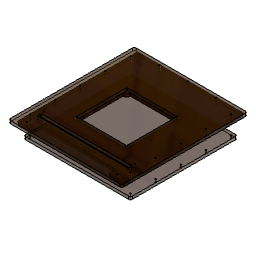
Module Plate Template (Autodesk Fusion 360 design; units mm, degrees)
Autodesk Fusion 360 part; units mm, degrees
sketch "Sketch1" plane through (0, 0, 0) normal (0, 0, 1) x (1, 0, 0)
  line L0 (-100, 0) -> (100, 0) construction
  line L1 (90, 0) -> (-90, 0)
  line L2 (-90, 0) -> (-90, 200)
  line L3 (-90, 200) -> (90, 200)
  line L4 (90, 200) -> (90, 0)
  line L5 (90, 0) -> (-90, 200) construction
  line L6 (-90, 0) -> (90, 200) construction
  line L7 (85, 0) -> (-85, 0)
  line L8 (-85, 0) -> (-85, 200)
  line L9 (-85, 200) -> (85, 200)
  line L10 (85, 200) -> (85, 0)
  line L11 (85, 0) -> (-85, 200) construction
  line L12 (-85, 0) -> (85, 200) construction
  line L13 (-60, 8) -> (-60, 21)
  line L14 (-60, 21) -> (60, 21)
  line L15 (60, 21) -> (60, 8)
  line L16 (60, 8) -> (-60, 21) construction
  line L17 (-60, 8) -> (60, 21) construction
  line L18 (-85, 8) -> (-60, 8)
  line L19 (60, 8) -> (85, 8)
  line L20 (0, 200) -> (0, 21) construction
  line L21 (40, 58) -> (-40, 58)
  line L22 (-40, 58) -> (-40, 138)
  line L23 (-40, 138) -> (40, 138)
  line L24 (40, 138) -> (40, 58)
  line L25 (40, 58) -> (-40, 138) construction
  line L26 (-40, 58) -> (40, 138) construction
  circle A0 centre (-40, 138) radius 1
  circle A1 centre (40, 138) radius 1
  circle A2 centre (-40, 58) radius 1
  circle A3 centre (40, 58) radius 1
  circle A4 centre (-40, 138) radius 6
  circle A5 centre (40, 138) radius 6
  circle A6 centre (40, 58) radius 6
  circle A7 centre (-40, 58) radius 6
  line L27 (-80, 200) -> (-80, 8) construction
  line L28 (80, 8) -> (80, 200) construction
  circle A8 centre (-80, 104) radius 1.1
  circle A9 centre (80, 104) radius 1.1
  circle A10 centre (80, 24) radius 1.1
  circle A11 centre (80, 64) radius 1.1
  circle A12 centre (80, 144) radius 1.1
  circle A13 centre (80, 184) radius 1.1
  circle A14 centre (-80, 24) radius 1.1
  circle A15 centre (-80, 64) radius 1.1
  circle A16 centre (-80, 144) radius 1.1
  circle A17 centre (-80, 184) radius 1.1
  line L29 (-85, 195) -> (85, 195) construction
  circle A18 centre (0, 195) radius 1.1
  circle A19 centre (-45, 195) radius 1.1
  circle A20 centre (45, 195) radius 1.1
  line L30 (85, 189) -> (-85, 189)
  line L31 (-85, 19) -> (85, 19)
  line L32 (72.5, 28) -> (-72.5, 28)
  line L33 (-72.5, 28) -> (-72.5, 34)
  line L34 (-72.5, 34) -> (72.5, 34)
  line L35 (72.5, 34) -> (72.5, 28)
  line L36 (72.5, 28) -> (-72.5, 34) construction
  line L37 (-72.5, 28) -> (72.5, 34) construction
  point P0 (0, 100)
  point P1 (0, 100)
  point P2 (0, 14.5)
  point P3 (0, 98)
  point P4 (0, 31)
  dimension "d2" = 200
  dimension "d7" = 180
  dimension "d8" = 170
  dimension "d9" = 200
  dimension "d12" = 8
  dimension "d18" = 120
  dimension "d19" = 13
  dimension "d20" = 80
  dimension "d21" = 80
  dimension "d22" = 2
  dimension "d23" = 2
  dimension "d24" = 2
  dimension "d25" = 2
  dimension "d27" = 12
  dimension "d28" = 12
  dimension "d29" = 12
  dimension "d30" = 12
  dimension "d38" = 5
  dimension "d39" = 5
  dimension "d41" = 2.2
  dimension "d44" = 0
  dimension "d45" = 80
  dimension "d46" = 2.2
  dimension "d49" = 0
  dimension "d50" = 80
  dimension "d52" = 50
  dimension "d55" = 5
  dimension "d56" = 2.2
  dimension "d59" = 45
  dimension "d60" = 0
  dimension "d61" = 5
  dimension "d62" = 5
  dimension "d77" = 145
  dimension "d78" = 6
  dimension "d79" = 31
  constraint horizontal L0
  constraint horizontal L1
  constraint perpendicular L1 L2
  constraint parallel L1 L3
  constraint parallel L2 L4
  constraint coincident L5 P1
  constraint coincident L6 P1
  constraint collinear L0 L1
  constraint horizontal L7
  constraint perpendicular L7 L8
  constraint parallel L7 L9
  constraint parallel L8 L10
  constraint coincident L11 P1
  constraint coincident L12 P1
  constraint coincident P1 P0
  constraint coincident L8 L18.start
  constraint coincident L10 L19.end
  constraint perpendicular L10 L18
  constraint parallel L13 L15
  constraint coincident L16 P2
  constraint coincident L17 P2
  constraint collinear L18 L19
  constraint midpoint L3 L20.start
  constraint midpoint L14 L20.end
  constraint perpendicular L14 L20
  constraint horizontal L21
  constraint perpendicular L21 L22
  constraint parallel L21 L23
  constraint parallel L22 L24
  constraint coincident L25 P3
  constraint coincident L26 P3
  constraint coincident L22.end L23.start
  constraint coincident L23.end L24.start
  constraint coincident L21.end L22.start
  constraint coincident L21.start L24.end
  constraint concentric A0 A4
  constraint concentric A1 A5
  constraint concentric A2 A7
  constraint coincident L18 L27.end
  constraint perpendicular L18 L27
  constraint coincident L19 L28.start
  constraint coincident L3 L28.end
  constraint midpoint L27 A8.centre
  constraint midpoint L28 A9.centre
  constraint coincident L20 P3
  constraint coincident L8 L29.start
  constraint coincident L10 L29.end
  constraint perpendicular L10 L29
  constraint midpoint L29 A18.centre
  constraint coincident L10 L30.start
  constraint coincident L8 L30.end
  constraint perpendicular L8 L30
  constraint coincident L8 L31.start
  constraint coincident L10 L31.end
  constraint perpendicular L10 L31
  constraint coincident L3 L27.start
  constraint horizontal L32
  constraint perpendicular L32 L33
  constraint parallel L32 L34
  constraint parallel L33 L35
  constraint coincident L36 P4
  constraint coincident L37 P4
  constraint coincident L20 P4
  measures "d2" distance of L1.end L2.end
  measures "d7" distance of L2.end L3.end
  measures "d8" distance of L8.end L9.end
  measures "d9" distance of L7.end L8.end
  measures "d12" distance of L7 L18
  measures "d18" distance of L13.end L14.end
  measures "d19" distance of L13.start L13.end
  measures "d20" distance of L21.end L22.end
  measures "d21" distance of L22.end L23.end
  measures "d22" diameter of A0
  measures "d23" diameter of A1
  measures "d24" diameter of A2
  measures "d25" diameter of A3
  measures "d27" diameter of A4
  measures "d28" diameter of A5
  measures "d29" diameter of A6
  measures "d30" diameter of A7
  measures "d38" distance of L10 L28
  measures "d39" distance of L8 L27
  measures "d41" diameter of A8
  measures "d46" diameter of A9
  measures "d52" distance of L19 L21
  measures "d55" distance of L3 L29
  measures "d56" diameter of A18
  measures "d61" distance of A13.centre L30
  measures "d62" distance of A10.centre L31
  measures "d77" distance of L33.end L34.end
  measures "d78" distance of L32.end L33.end
  measures "d79" distance of L0 P4
extrude "Extrude1" add sketch "Sketch1" along normal blind 4.5 contours L1 L3 L4 L10 | L1 L7 L8 L10 L13 L15 L18 L19 L31 | L1 L2 L3 L8 | L10 L15 L19 L31 | L3 L8 L9 L10 L30 | L8 L13 L18 L31 | L8 L10 L13 L14 L15 L30 L31 | L13 L14 L15 L31 | L21 L22 A2 A7 | L21 L24 A3 A6 | L22 L23 A0 A4 | L23 L24 A1 A5 picked at (-39.2853, 53.7378) picked at (35.689, 57.7019) picked at (-44.0958, 136.6211) picked at (36.2453, 140.139) makes body 1
extrude "Extrude2" add sketch "Sketch1" against normal blind 4.5 separate body contours L10 L15 L19 L31 | L3 L8 L9 L10 L30 | L8 L13 L18 L31 | L8 L10 L13 L14 L15 L30 L31 | L21 L22 A2 A7 | L21 L22 A2 A7 | L21 L22 A2 | L21 L22 A2 | L21 L24 A3 A6 | L21 L24 A3 A6 | L21 L24 A3 | L21 L24 A3 | L22 L23 A0 A4 | L22 L23 A0 A4 | L23 L24 A1 A5 | L23 L24 A1 A5 | L22 L23 A0 | L22 L23 A0 | L23 L24 A1 | L23 L24 A1 makes body 2
fillet "Fillet1" radius 3 10 edges at (90, 0, 2.25) (-90, 0, 2.25) (90, 200, 2.25) (-90, 200, 2.25) (85, 8, -2.25) (-85, 8, -2.25) (-60, 8, -2.25) (60, 8, -2.25) (85, 200, -2.25) (-85, 200, -2.25) on bodies 1 2
fillet "Fillet2" radius 1 2 edges at (60, 21, -2.25) (-60, 21, -2.25) on bodies 2
extrude "Extrude3" add sketch "Sketch1" against normal blind 4.5 from surface at -4.5 separate body contours L8 L10 L13 L14 L15 L30 L31 | L13 L14 L15 L31 | L21 L22 A2 A7 | L21 L22 L23 L24 A4 A5 A6 A7 | L21 L22 A2 A7 | L21 L22 A2 | L21 L22 A2 | L21 L24 A3 A6 | L21 L24 A3 A6 | L21 L24 A3 | L21 L24 A3 | L22 L23 A0 A4 | L22 L23 A0 A4 | L23 L24 A1 A5 | L23 L24 A1 A5 | L22 L23 A0 | L22 L23 A0 | L23 L24 A1 | L23 L24 A1 | L32 L33 L34 L35 makes body 3
fillet "Fillet3" radius 3 4 edges at (85, 189, -6.75) (85, 19, -6.75) (-85, 19, -6.75) (-85, 189, -6.75) on bodies 3
move_body "Move1" bodies 3 to x (1, 0, 0) y (0, 1, 0) z (0, 0, 1) at (0, 0, -16)
sketch "Sketch2" plane through (0, 0, 4.5) normal (0, 0, 1) x (-1, 0, 0)
  arc A0 (87, -200) -> (90, -197) centre (87, -197) ccw
  line L0 (90, -197) -> (90, -3)
  arc A1 (90, -3) -> (87, 0) centre (87, -3) ccw
  line L1 (87, 0) -> (-87, 0)
  arc A2 (-87, 0) -> (-90, -3) centre (-87, -3) ccw
  line L2 (-90, -3) -> (-90, -197)
  arc A3 (-90, -197) -> (-87, -200) centre (-87, -197) ccw
  line L3 (-87, -200) -> (87, -200)
  circle A4 centre (-80, -104) radius 1.1
  circle A5 centre (-80, -184) radius 1.1
  circle A6 centre (-80, -64) radius 1.1
  circle A7 centre (45, -195) radius 1.1
  circle A8 centre (80, -144) radius 1.1
  circle A9 centre (-45, -195) radius 1.1
  circle A10 centre (80, -104) radius 1.1
  circle A11 centre (0, -195) radius 1.1
  circle A12 centre (80, -184) radius 1.1
  circle A13 centre (80, -24) radius 1.1
  circle A14 centre (-80, -144) radius 1.1
  circle A15 centre (80, -64) radius 1.1
  circle A16 centre (-80, -24) radius 1.1
  arc A17 (40, -59) -> (39, -58) centre (40, -58) ccw
  line L4 (40, -59) -> (40, -137)
  arc A18 (39, -138) -> (40, -137) centre (40, -138) ccw
  line L5 (39, -138) -> (-39, -138)
  arc A19 (-40, -137) -> (-39, -138) centre (-40, -138) ccw
  line L6 (-40, -137) -> (-40, -59)
  arc A20 (-39, -58) -> (-40, -59) centre (-40, -58) ccw
  line L7 (-39, -58) -> (39, -58)
  line L8 (-72, -11) -> (72, -11) construction
  line L9 (72, -11) -> (72, -39) construction
  line L10 (72, -39) -> (-72, -39) construction
  line L11 (-72, -39) -> (-72, -11) construction
  line L12 (-72, -11) -> (72, -39) construction
  line L13 (72, -11) -> (-72, -39) construction
  line L14 (-95, 0) -> (95, 0) construction
  line L15 (0, 10) -> (0, -210) construction
  circle A21 centre (-72, -39) radius 1.1
  circle A22 centre (-72, -11) radius 1.1
  circle A23 centre (72, -39) radius 1.1
  circle A24 centre (72, -11) radius 1.1
  line L16 (72.5, -34) -> (-72.5, -34)
  line L17 (-72.5, -34) -> (-72.5, -28)
  line L18 (-72.5, -28) -> (72.5, -28)
  line L19 (72.5, -28) -> (72.5, -34)
  point P0 (0, -25)
  dimension "d68" = 28
  dimension "d69" = 144
  dimension "d70" = 11
  dimension "d71" = 2.2
  dimension "d72" = 2.2
  dimension "d73" = 2.2
  dimension "d74" = 2.2
  constraint horizontal L8
  constraint perpendicular L8 L9
  constraint parallel L8 L10
  constraint parallel L9 L11
  constraint coincident L12 P0
  constraint coincident L13 P0
  constraint parallel L1 L14
  constraint perpendicular L1 L15
  constraint coincident P0 L15
  constraint coincident L10.end L11.start
  constraint coincident L8.start L11.end
  constraint coincident L9.end L10.start
  constraint coincident L8.end L9.start
  measures "d68" distance of L8.end L9.end
  measures "d69" distance of L9.end L10.end
  measures "d70" distance of L8 L14
  measures "d71" diameter of A21
  measures "d72" diameter of A22
  measures "d73" diameter of A23
  measures "d74" diameter of A24
extrude "Extrude4" cut sketch "Sketch2" against normal blind 9 contours A21 | A22 | A23 | A24 bodies 1 2
fillet "Fillet4" radius 1 8 edges at (-72.5, 28, 2.25) (-72.5, 34, 2.25) (72.5, 34, 2.25) (72.5, 28, 2.25) (-72.5, 28, -2.25) (-72.5, 34, -2.25) (72.5, 34, -2.25) (72.5, 28, -2.25) on bodies 1 2
move_body "Move2" bodies 3 to x (1, 0, 0) y (0, 1, 0) z (0, 0, 1) at (0, 0, -2)
move_body "Move3" bodies 3 to x (1, 0, 0) y (0, 1, 0) z (0, 0, 1) at (0, 0, -2)
equation "d2 = ModuleLength"
equation "ModuleLength = 200 mm"
equation "ModuleWidth = 180 mm"
equation "DUTWidth = 80 mm"
equation "DUTLength = 80 mm"
equation "d7 = ModuleWidth"
equation "d8 = ModuleWidth - 10 mm"
equation "d9 = ModuleLength"
equation "CornerRelief = 2 mm"
equation "d20 = DUTLength"
equation "d21 = DUTWidth"
equation "d22 = CornerRelief"
equation "d23 = CornerRelief"
equation "d24 = CornerRelief"
equation "d25 = CornerRelief"
equation "CornerSupport = 12 mm"
equation "d27 = CornerSupport"
equation "d28 = CornerSupport"
equation "d29 = CornerSupport"
equation "d30 = CornerSupport"
equation "CornerFillet = 3 mm"
equation "d37 = CornerFillet"
equation "BoltHole = 2.2 mm"
equation "d41 = BoltHole"
equation "d45 = ModuleLength / 2.5"
equation "d46 = BoltHole"
equation "d50 = ModuleLength / 2.5"
equation "DUTFrontOffset = 50 mm"
equation "d52 = DUTFrontOffset"
equation "d56 = BoltHole"
equation "d59 = ModuleWidth / 4"
named bodies: "Top Plate", "Base Plate", "Support Plate"
